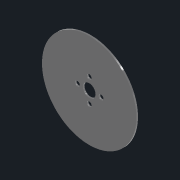
# Autodesk Inventor part: plate
Saved by Autodesk Inventor 2022.2 (Build 262287010, 287A)
## iProperties
Created: 2023-07-21
Part Number: plate
Material: Steel
Document SubType Name: Modeling
Designer: StijnC
Density: 7.85 g/cm^3
Appearance: Silicon Nitride - Polished
Author: StijnC
Autodesk Inventor part; units mm, degrees
ref_plane "YZ Plane" through (0, 0, 0) normal (1, 0, 0) x (0, 1, 0)
ref_plane "XZ Plane" through (0, 0, 0) normal (0, 1, 0) x (-1, 0, 0)
ref_plane "XY Plane" through (0, 0, 0) normal (0, 0, 1) x (1, 0, 0)
sketch "Sketch1" plane through (0, 0, 0) normal (0, 0, 1) x (1, 0, 0)
  circle A0 centre (0, 0) radius 30
  dimension "d0" = 60
  constraints: 1 centre point, 1 coincident
  measures "d0" diameter of A0
extrude "Extrusion1" add sketch "Sketch1" along normal mid plane 1
sketch "Sketch2" plane through (0, 0, 0.5) normal (0, 0, 1) x (1, 0, 0)
  point P0 (0, 0)
  point P1 (0, 0)
  constraints: 1 coincident
hole "Hole1" at (0, 0, 0.5) direction (0, 0, -1) diameter 8 end through all
sketch "Sketch3" plane through (0, 0, 0.5) normal (0, 0, 1) x (1, 0, 0)
  circle A0 centre (0, 0) radius 4 projected
  circle A1 centre (0, 0) radius 7.5 construction
  point P0 (-7.5, 0)
  point P1 (0, 7.5)
  point P2 (7.5, 0)
  point P3 (0, -7.5)
  dimension "d10" = 15
  constraints: 4 point on circle, 2 horizontal alignment, 2 vertical alignment, 1 centre point, 1 coincident
  measures "d10" diameter of A1
hole "Hole2" at (-7.5, 0, 0.5) at (0, 7.5, 0.5) at (7.5, 0, 0.5) at (0, -7.5, 0.5) direction (0, 0, -1) diameter 3 end through all
body "Solid1"
